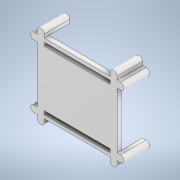
# Autodesk Inventor part: cover
Saved by Autodesk Inventor 2020 (Build 240168000, 168)
## iProperties
Created: 2019-06-14
Part Number: cover
Material: ABS Plastic
Document SubType Name: Modeling
Designer: amirt
Density: 1.06 g/cm^3
Appearance: Smooth - White
Author: amirt
Autodesk Inventor part; units mm, degrees
ref_plane "YZ Plane" through (0, 0, 0) normal (1, 0, 0) x (0, 1, 0)
ref_plane "XZ Plane" through (0, 0, 0) normal (0, 1, 0) x (-1, 0, 0)
ref_plane "XY Plane" through (0, 0, 0) normal (0, 0, 1) x (1, 0, 0)
ref_plane "Work Plane1" through (1.3068, 17.1014, 0) normal (0, 0, 1) x (1, 0, 0)
sketch "Sketch2" plane through (1.3068, 17.1014, 0) normal (0, 0, 1) x (1, 0, 0)
  line L0 (-22, -19.25) -> (-22, 19.25)
  line L1 (-22, 19.25) -> (22, 19.25)
  line L2 (22, -19.25) -> (-22, -19.25)
  line L3 (-22, 19.25) -> (22, 19.25)
  line L4 (22, 19.25) -> (22, -19.25)
  line L5 (-22, 19.25) -> (22, 19.25)
  line L6 (-22, 19.25) -> (-18.19, 19.25)
  line L7 (-18.19, 19.25) -> (-18.19, 21.155)
  line L8 (-20.095, 23.06) -> (-20.095, 23.06)
  line L9 (-22, 21.155) -> (-22, 19.25)
  line L10 (-22, 19.25) -> (-23.905, 19.25)
  line L11 (-25.81, 17.345) -> (-25.81, 17.345)
  line L12 (-23.905, 15.44) -> (-22, 15.44)
  line L13 (-22, 15.44) -> (-22, 19.25)
  line L14 (-22, -19.25) -> (-23.905, -19.25)
  line L15 (-25.81, -17.345) -> (-25.81, -17.345)
  line L16 (-23.905, -15.44) -> (-22, -15.44)
  line L17 (-22, -15.44) -> (-22, -19.25)
  line L18 (-22, -19.25) -> (-18.19, -19.25)
  line L19 (-18.19, -19.25) -> (-18.19, -21.155)
  line L20 (-20.095, -23.06) -> (-20.095, -23.06)
  line L21 (-22, -21.155) -> (-22, -19.25)
  line L22 (22, -19.25) -> (18.19, -19.25)
  line L23 (18.19, -19.25) -> (18.19, -21.155)
  line L24 (20.095, -23.06) -> (20.095, -23.06)
  line L25 (22, -21.155) -> (22, -19.25)
  line L26 (22, -19.25) -> (23.905, -19.25)
  line L27 (25.81, -17.345) -> (25.81, -17.345)
  line L28 (23.905, -15.44) -> (22, -15.44)
  line L29 (22, -15.44) -> (22, -19.25)
  line L30 (22, 19.25) -> (23.905, 19.25)
  line L31 (25.81, 17.345) -> (25.81, 17.345)
  line L32 (23.905, 15.44) -> (22, 15.44)
  line L33 (22, 15.44) -> (22, 19.25)
  line L34 (22, 19.25) -> (18.19, 19.25)
  line L35 (18.19, 19.25) -> (18.19, 21.155)
  line L36 (20.095, 23.06) -> (20.095, 23.06)
  line L37 (22, 21.155) -> (22, 19.25)
  arc A0 (22, 21.155) -> (20.095, 23.06) centre (20.095, 21.155) ccw
  arc A1 (25.81, 17.345) -> (23.905, 19.25) centre (23.905, 17.345) ccw
  arc A2 (23.905, 15.44) -> (25.81, 17.345) centre (23.905, 17.345) ccw
  arc A3 (20.095, 23.06) -> (18.19, 21.155) centre (20.095, 21.155) ccw
  arc A4 (23.905, -19.25) -> (25.81, -17.345) centre (23.905, -17.345) ccw
  arc A5 (25.81, -17.345) -> (23.905, -15.44) centre (23.905, -17.345) ccw
  arc A6 (20.095, -23.06) -> (22, -21.155) centre (20.095, -21.155) ccw
  arc A7 (18.19, -21.155) -> (20.095, -23.06) centre (20.095, -21.155) ccw
  arc A8 (-22, -21.155) -> (-20.095, -23.06) centre (-20.095, -21.155) ccw
  arc A9 (-20.095, -23.06) -> (-18.19, -21.155) centre (-20.095, -21.155) ccw
  arc A10 (-25.81, -17.345) -> (-23.905, -19.25) centre (-23.905, -17.345) ccw
  arc A11 (-23.905, -15.44) -> (-25.81, -17.345) centre (-23.905, -17.345) ccw
  arc A12 (-25.81, 17.345) -> (-23.905, 15.44) centre (-23.905, 17.345) ccw
  arc A13 (-23.905, 19.25) -> (-25.81, 17.345) centre (-23.905, 17.345) ccw
  arc A14 (-20.095, 23.06) -> (-22, 21.155) centre (-20.095, 21.155) ccw
  arc A15 (-18.19, 21.155) -> (-20.095, 23.06) centre (-20.095, 21.155) ccw
  line L38 (18.19, 17.345) -> (-18.19, 17.345)
  line L39 (-18.19, 17.345) -> (-18.19, 15.44)
  line L40 (-18.19, 15.44) -> (18.19, 15.44)
  line L41 (18.19, 15.44) -> (18.19, 17.345)
  line L42 (18.19, -17.345) -> (-18.19, -17.345)
  line L43 (-18.19, -17.345) -> (-18.19, -15.44)
  line L44 (-18.19, -15.44) -> (18.19, -15.44)
  line L45 (18.19, -15.44) -> (18.19, -17.345)
  point P0 (-1.3068, -17.1014)
  point P1 (0, 0)
  point P2 (-18.19, 23.06)
  point P3 (-22, 23.06)
  point P4 (-25.81, 15.44)
  point P5 (-25.81, 19.25)
  point P6 (-25.81, -15.44)
  point P7 (-25.81, -19.25)
  point P8 (-18.19, -23.06)
  point P9 (-22, -23.06)
  point P10 (18.19, -23.06)
  point P11 (22, -23.06)
  point P12 (25.81, -15.44)
  point P13 (25.81, -19.25)
  point P14 (25.81, 15.44)
  point P15 (25.81, 19.25)
  point P16 (18.19, 23.06)
  point P17 (22, 23.06)
  point P18 (-20.095, -23.06)
  dimension "d21" = 3.81
  dimension "d22" = 3.81
  dimension "d23" = 3.81
  dimension "d24" = 3.81
  dimension "d25" = 3.81
  dimension "d26" = 3.81
  dimension "d27" = 3.81
  dimension "d28" = 3.81
  dimension "d29" = 3.81
  dimension "d30" = 3.81
  dimension "d31" = 3.81
  dimension "d32" = 3.81
  dimension "d33" = 3.81
  dimension "d34" = 3.81
  dimension "d35" = 3.81
  dimension "d36" = 3.81
  dimension "d37" = 1.905
  dimension "d38" = 1.905
  dimension "d39" = 1.905
  constraints: 92 end point, 34 point on line, 32 point on circle, 32 tangent, 20 parallel, 16 centre point, 13 equal radius, 10 horizontal, 10 perpendicular
  measures "d21" distance of point (-22, 23.06) point (-18.19, 23.06)
  measures "d22" distance of point (-18.19, 23.06) L7.start
  measures "d23" distance of L13.start point (-25.81, 15.44)
  measures "d24" distance of point (-25.81, 15.44) point (-25.81, 19.25)
  measures "d25" distance of point (-25.81, -15.44) L17.start
  measures "d26" distance of point (-25.81, -19.25) point (-25.81, -15.44)
  measures "d27" distance of point (-18.19, -23.06) point (-22, -23.06)
  measures "d28" distance of L18.end point (-18.19, -23.06)
  measures "d29" distance of point (22, -23.06) point (18.19, -23.06)
  measures "d30" distance of point (18.19, -23.06) L22.end
  measures "d31" distance of L29.start point (25.81, -15.44)
  measures "d32" distance of point (25.81, -15.44) point (25.81, -19.25)
  measures "d33" distance of point (25.81, 15.44) L33.start
  measures "d34" distance of point (25.81, 19.25) point (25.81, 15.44)
  measures "d35" distance of point (18.19, 23.06) point (22, 23.06)
  measures "d36" distance of L35.start point (18.19, 23.06)
  measures "d37" radius of A0
  measures "d38" radius of A2
  measures "d39" radius of A6
extrude "Extrusion2" add sketch "Sketch2" along normal blind 2.54
sketch "Sketch4" plane through (1.3068, 17.1014, 0) normal (0, 0, -1) x (-1, 0, 0)
  line L0 (22, 21.155) -> (22, 19.25) projected
  arc A0 (22, 21.155) -> (18.19, 21.155) centre (20.095, 21.155) ccw projected
  line L1 (18.19, 19.25) -> (18.19, 21.155) projected
  line L2 (22, 19.25) -> (23.905, 19.25) projected
  arc A1 (23.905, 15.44) -> (23.905, 19.25) centre (23.905, 17.345) ccw projected
  line L3 (23.905, 15.44) -> (22, 15.44) projected
  line L4 (-23.905, 19.25) -> (-22, 19.25) projected
  arc A2 (-23.905, 19.25) -> (-23.905, 15.44) centre (-23.905, 17.345) ccw projected
  line L5 (-22, 15.44) -> (-23.905, 15.44) projected
  line L6 (-22, 19.25) -> (-22, 21.155) projected
  arc A3 (-18.19, 21.155) -> (-22, 21.155) centre (-20.095, 21.155) ccw projected
  line L7 (-18.19, 21.155) -> (-18.19, 19.25) projected
  line L8 (-23.905, -15.44) -> (-22, -15.44) projected
  arc A4 (-23.905, -15.44) -> (-23.905, -19.25) centre (-23.905, -17.345) ccw projected
  line L9 (-22, -19.25) -> (-23.905, -19.25) projected
  line L10 (-22, -21.155) -> (-22, -19.25) projected
  arc A5 (-22, -21.155) -> (-18.19, -21.155) centre (-20.095, -21.155) ccw projected
  line L11 (-18.19, -19.25) -> (-18.19, -21.155) projected
  line L12 (18.19, -21.155) -> (18.19, -19.25) projected
  arc A6 (18.19, -21.155) -> (22, -21.155) centre (20.095, -21.155) ccw projected
  line L13 (22, -19.25) -> (22, -21.155) projected
  line L14 (23.905, -19.25) -> (22, -19.25) projected
  line L15 (22, -15.44) -> (23.905, -15.44) projected
  arc A7 (23.905, -19.25) -> (23.905, -15.44) centre (23.905, -17.345) ccw projected
  line L16 (22, -15.44) -> (22, -19.25)
  line L17 (18.19, -19.25) -> (22, -19.25)
  line L18 (-22, -19.25) -> (-18.19, -19.25)
  line L19 (-22, -15.44) -> (-22, -19.25)
  line L20 (-22, 19.25) -> (-22, 15.44)
  line L21 (-22, 19.25) -> (-18.19, 19.25)
  line L22 (18.19, 19.25) -> (22, 19.25)
  line L23 (22, 21.155) -> (22, 19.25) projected
  line L24 (22, 15.44) -> (22, 19.25)
  point P0 (1.3068, -17.1014)
  constraints: 16 end point, 3 perpendicular, 2 collinear, 2 vertical, 1 horizontal
extrude "Extrusion3" add sketch "Sketch4" along normal blind 11.545
body "Solid1"
